Autodesk Fusion 360 part; units mm, degrees
(part 2 of 2)
sketch "Sketch6 (2)" plane through (0, -47, 0) normal (0, -1, 0) x (1, 0, 0) in component "DoserBase"
  line L0 (61.125, -2.25) -> (56.75, -2.25)
  line L1 (56.75, -2.25) -> (56.75, -6.75)
  line L2 (56.75, -6.75) -> (33, -6.75)
  line L3 (33, -6.75) -> (33, 6.75)
  line L4 (33, 6.75) -> (20, 6.75)
  line L5 (20, 6.75) -> (20, 20)
  line L6 (20, 20) -> (-10, 20)
  line L7 (-10, 20) -> (-10, -20)
  line L8 (-10, -20) -> (20, -20)
  line L9 (20, -20) -> (20, -11.75)
  line L10 (20, -11.75) -> (61.125, -11.75)
  line L11 (61.125, -11.75) -> (61.125, -2.25)
  line L12 (-7, 17) -> (17, 17)
  line L13 (17, 17) -> (17, -17)
  line L14 (17, -17) -> (-7, -17)
  line L15 (-7, -17) -> (-7, 17)
  line L16 (17, 3.75) -> (30, 3.75)
  line L17 (30, 3.75) -> (30, -8.75)
  line L18 (30, -8.75) -> (17, -8.75)
  line L19 (26.5, 15) -> (26.5, -15) construction
  line L20 (-10, 0) -> (26.5, 0) construction
  circle A0 centre (26.5, -15) radius 1.75
  circle A1 centre (26.5, 15) radius 1.75
  line L21 (20, 20) -> (33, 20)
  line L22 (33, 20) -> (33, 6.75)
  line L23 (20, -20) -> (33, -20)
  line L24 (33, -20) -> (33, -11.75)
  line L25 (33, -6.75) -> (33, -11.75) construction
  line L26 (26.5, 15) -> (26.5, 20) construction
  line L27 (-10, 20) -> (-17, 20)
  line L28 (-17, 20) -> (-17, -20)
  line L29 (-17, -20) -> (-10, -20)
  line L30 (-13.5, 20) -> (-13.5, -20) construction
  line L31 (26.5, 15) -> (-13.5, 15) construction
  line L32 (26.5, -15) -> (-13.5, -15) construction
  circle A2 centre (-13.5, 15) radius 1.75
  circle A3 centre (-13.5, -15) radius 1.75
  dimension "d242" = 3
  dimension "d243" = 3
  dimension "d244" = 3
  dimension "d245" = 3
  dimension "d246" = 3
  dimension "d247" = 3
  dimension "d248" = 3
  dimension "d254" = 30
  dimension "d257" = 3.5
  dimension "d258" = 3.5
  dimension "d260" = 3.5
  dimension "d261" = 3.5
  dimension "d262" = 40
  constraint horizontal L12
  constraint vertical L13
  constraint horizontal L14
  constraint vertical L15
  constraint coincident L13 L16.start
  constraint perpendicular L13 L16
  constraint perpendicular L16 L17
  constraint coincident L13 L18.end
  constraint perpendicular L13 L18
  constraint vertical L19
  constraint midpoint L7 L20.start
  constraint midpoint L19 L20.end
  constraint horizontal L20
  constraint coincident L19.end A0.centre
  constraint coincident L19.start A1.centre
  constraint coincident L5.end L6.start
  constraint perpendicular L5 L21
  constraint coincident L3.end L4.start
  constraint perpendicular L21 L22
  constraint coincident L8.end L9.start
  constraint perpendicular L9 L23
  constraint coincident L10 L24.end
  constraint perpendicular L10 L24
  constraint coincident L2.end L3.start
  constraint vertical L25
  constraint midpoint L21 L26.end
  constraint vertical L26
  constraint coincident L6.end L7.start
  constraint perpendicular L7 L27
  constraint perpendicular L27 L28
  constraint coincident L7.end L8.start
  constraint perpendicular L28 L29
  constraint midpoint L27 L30.start
  constraint midpoint L29 L30.end
  constraint coincident L30 L31.end
  constraint perpendicular L30 L31
  constraint coincident L30 L32.end
  constraint perpendicular L30 L32
  constraint coincident L31.end A2.centre
  constraint coincident L32.end A3.centre
  measures "d242" distance of L9 L13
  measures "d243" distance of L8 L14
  measures "d244" distance of L7 L15
  measures "d245" distance of L6 L12
  measures "d246" distance of L10 L18
  measures "d247" distance of L4 L16
  measures "d248" distance of L3 L17
  measures "d254" distance of L19.start L19.end
  measures "d257" diameter of A1
  measures "d258" diameter of A0
  measures "d260" diameter of A3
  measures "d261" diameter of A2
  measures "d262" distance of L19.start L31.end
extrude "Extrude11" cut sketch "Sketch6 (2)" against normal blind 43 contours L12 L13 L14 L15 bodies 2 in component "DoserBase"
extrude "Extrude12" cut sketch "Sketch6 (2)" against normal blind 21 contours L13 L16 L17 L18 bodies 2 in component "DoserBase"
chamfer "Chamfer2'" distance 1 angle 45 2 edges at (20, -33.15, -11.75) (20, -33.15, 6.75) on bodies 2 in component "DoserBase"
extrude "Extrude13" add sketch "Sketch6 (2)" against normal blind 3 contours L9 L10 L23 L24 | L4 L5 L21 L22 | L7 L27 L28 L29 bodies 2 in component "DoserBase"
sketch "Sketch8" plane through (-10, 0, 0) normal (-1, 0, 0) x (0, 0, 1) in component "DoserBase"
  line L0 (-20, -44) -> (20, -44)
  line L1 (20, -44) -> (20, 10.5)
  line L2 (20, 10.5) -> (11.5, 10.5)
  line L3 (11.5, 10.5) -> (11.5, 0)
  line L4 (11.5, 0) -> (-11.5, 0)
  line L5 (-11.5, 0) -> (-11.5, 10.5)
  line L6 (-11.5, 10.5) -> (-20, 10.5)
  line L7 (-20, 10.5) -> (-20, -44)
  line L8 (-20, -10) -> (20, -10) construction
  line L9 (-12.5, -5) -> (12.5, -5) construction
  line L10 (12.5, -5) -> (12.5, -15) construction
  line L11 (12.5, -15) -> (-12.5, -15) construction
  line L12 (-12.5, -15) -> (-12.5, -5) construction
  circle A0 centre (-12.5, -15) radius 0.75
  circle A1 centre (-12.5, -5) radius 0.75
  circle A2 centre (12.5, -5) radius 0.75
  circle A3 centre (12.5, -15) radius 0.75
  line L13 (0, -5) -> (0, 0) construction
  dimension "d265" = 10
  dimension "d266" = 1.5
  dimension "d267" = 1.5
  dimension "d268" = 1.5
  dimension "d269" = 1.5
  dimension "d270" = 10
  dimension "d271" = 25
  dimension "d272" = 5
  constraint coincident L7 L8.start
  constraint coincident L1 L8.end
  constraint perpendicular L1 L8
  constraint horizontal L9
  constraint vertical L10
  constraint horizontal L11
  constraint vertical L12
  constraint coincident L11.end L12.start
  constraint coincident L9.start L12.end
  constraint coincident L9.end L10.start
  constraint coincident L10.end L11.start
  constraint midpoint L9 L13.start
  constraint coincident L13.end origin
  constraint vertical L13
  measures "d265" distance of L4 L8
  measures "d266" diameter of A1
  measures "d267" diameter of A0
  measures "d268" diameter of A2
  measures "d269" diameter of A3
  measures "d270" distance of L9.start L11.end
  measures "d271" distance of L10.end L11.end
  measures "d272" distance of L8 L9
extrude "Extrude14" cut sketch "Sketch8" against normal up to surface (3 mm away) contours A0 | A1 | A2 | A3 bodies 2 in component "DoserBase"
sketch "Sketch1 (9)" plane through (-10, 0, 0) normal (-1, 0, 0) x (0, 0, 1) in component "Shoot"
  circle A0 centre (-12.5, -15) radius 0.75
  circle A1 centre (-12.5, -5) radius 0.75
  circle A2 centre (12.5, -15) radius 0.75
  circle A3 centre (12.5, -5) radius 0.75
  line L0 (-20, -44) -> (20, -44)
  line L1 (20, -44) -> (20, 10.5)
  line L2 (20, 10.5) -> (11.5, 10.5)
  line L3 (11.5, 10.5) -> (11.5, 0)
  line L4 (11.5, 0) -> (-11.5, 0)
  line L5 (-11.5, 0) -> (-11.5, 10.5)
  line L6 (-11.5, 10.5) -> (-20, 10.5)
  line L7 (-20, 10.5) -> (-20, -44)
  line L8 (-14.5, -3) -> (14.5, -3)
  line L9 (14.5, -3) -> (14.5, -17)
  line L10 (14.5, -17) -> (-14.5, -17)
  line L11 (-14.5, -17) -> (-14.5, -3)
  circle A4 centre (-12.5, -5) radius 1
  circle A5 centre (-12.5, -15) radius 1
  circle A6 centre (12.5, -15) radius 1
  circle A7 centre (12.5, -5) radius 1
  line L12 (-12.5, -5) -> (12.5, -15) construction
  line L13 (-14.5, -17) -> (14.5, -3) construction
  dimension "d279" = 2
  dimension "d280" = 2
  dimension "d281" = 2
  dimension "d282" = 2
  dimension "d283" = 14
  dimension "d284" = 29
  constraint horizontal L8
  constraint vertical L9
  constraint horizontal L10
  constraint vertical L11
  constraint concentric A1 A4
  constraint concentric A0 A5
  constraint concentric A2 A6
  constraint concentric A3 A7
  constraint coincident A1.centre A4.centre
  constraint coincident A2.centre A6.centre
  constraint midpoint L12 L13
  measures "d279" diameter of A4
  measures "d280" diameter of A5
  measures "d281" diameter of A6
  measures "d282" diameter of A7
  measures "d283" distance of L8.end L9.end
  measures "d284" distance of L9.end L10.end
extrude "Extrude1''''''''" add sketch "Sketch1 (9)" along normal blind 2 separate body contours L8 L9 L10 L11 makes body 23 in component "Shoot"
ref_plane "WorkPlane1" through (-11, -10, 0) normal (0, 1, 0) x (0, 0, -1) in component "Shoot"
sketch "Sketch3 (6)" plane through (0, -10, 0) normal (0, 1, 0) x (1, 0, 0) in component "Shoot"
  circle A0 centre (-20.25, 0) radius 8.5 construction
  circle A1 centre (-28.5, 40) radius 10
  circle A2 centre (-20.25, 0) radius 10
  line L0 (-30.0439, -2.02) -> (-38.2939, 37.98)
  line L1 (-18.7061, 42.02) -> (-10.4561, 2.02)
  line L2 (-12, -14.5) -> (-12, 14.5)
  line L3 (-12, -10) -> (-20.25, -10)
  line L4 (-10, -14.5) -> (-10, 14.5)
  line L5 (-10, 14.5) -> (-10, 50)
  line L6 (-10, 50) -> (-28.5, 50)
  line L7 (-12, -10) -> (-10, -10)
  arc A3 (-20.5, 40) -> (-36.5, 40) centre (-28.5, 40) ccw construction
  dimension "d287" = 20
  dimension "d288" = 20
  constraint concentric A1 A3
  constraint concentric A0 A2
  constraint coincident A2 L0.start
  constraint coincident A1 L0.end
  constraint tangent A1 L0
  constraint coincident A1 L1.start
  constraint coincident A2 L1.end
  constraint tangent A2 L1
  constraint tangent A2 L0
  constraint tangent A1 L1
  constraint coincident L2 L3.start
  constraint coincident A2 L3.end
  constraint tangent A2 L3
  constraint horizontal L3
  constraint coincident L4.end L5.start
  constraint parallel L4 L5
  constraint coincident A1 L6.end
  constraint tangent A1 L6
  constraint perpendicular L5 L6
  constraint coincident L4 L7.end
  constraint perpendicular L4 L7
  measures "d287" diameter of A1
  measures "d288" diameter of A2
extrude "Extrude2'''''''" add sketch "Sketch3 (6)" along normal blind -12 and the other way blind -2 bodies 23 in component "Shoot"
sketch "Sketch4 (5)" plane through (-12, 0, 0) normal (-1, 0, 0) x (0, 0, 1) in component "Shoot"
  line L0 (-14.5, -8) -> (10, -8) construction
  line L1 (10, -8) -> (10, -17) construction
  line L2 (10, -17) -> (14.5, -17) construction
  line L3 (14.5, -17) -> (14.5, -3)
  line L4 (14.5, -3) -> (-14.5, -3)
  line L5 (-14.5, -3) -> (-14.5, -8) construction
  circle A0 centre (12.5, -5) radius 1 construction
  circle A1 centre (12.5, -15) radius 1 construction
  circle A2 centre (-12.5, -5) radius 1 construction
  line L6 (14.5, -6.8072) -> (-31.5, -19)
  line L7 (-31.5, -19) -> (-30.2189, -23.8331)
  line L8 (-30.2189, -23.8331) -> (14.5, -11.9799)
  line L9 (2.02, -8) -> (-37.98, -8)
  line L10 (14.5, -17) -> (14.5, -53)
  line L11 (14.5, -53) -> (-85.5, -53)
  line L12 (-85.5, -53) -> (-85.5, -3)
  line L13 (-85.5, -3) -> (-14.5, -3)
  point P0 (10, -8)
  dimension "d291" = 5
  dimension "d292" = 17
  dimension "d293" = 11
  dimension "d294" = 100
  dimension "d295" = 50
  constraint perpendicular L6 L7
  constraint coincident L3 L8.end
  constraint perpendicular L7 L8
  constraint coincident L3 L6.start
  constraint coincident L6 P0
  constraint coincident L2.end L3.start
  constraint perpendicular L2 L10
  constraint perpendicular L10 L11
  constraint perpendicular L11 L12
  constraint coincident L4.end L5.start
  constraint perpendicular L12 L13
  measures "d291" distance of L6.end L7.end
  measures "d292" distance of L5 L6.end
  measures "d293" distance of L6.end L9
  measures "d294" distance of L10.end L11.end
  measures "d295" distance of L11.end L12.end
extrude "Extrude3'''" cut sketch "Sketch4 (5)" along normal blind 30 contours L3 L4 L6 L7 L8 L10 L11 L12 L13 bodies 23 in component "Shoot"
sketch "Sketch6 (3)" plane through (-10, 0, 0) normal (1, 0, 0) x (0, 0, -1) in component "Shoot"
  line L0 (-10, -22) -> (50, -22)
  line L1 (50, -22) -> (50, -8)
  line L2 (50, -8) -> (14.5, -8)
  line L3 (14.5, -8) -> (14.5, -3)
  line L4 (14.5, -3) -> (-14.5, -3)
  line L5 (-14.5, -3) -> (-14.5, -17)
  circle A0 centre (-12.5, -5) radius 1
  circle A1 centre (-12.5, -15) radius 1
  circle A2 centre (12.5, -5) radius 1
  line L6 (31.5, -19) -> (30.7048, -22)
  line L7 (14.5, -8) -> (14.5, -14.494)
  line L8 (-10, -8) -> (31.5, -19)
  line L9 (-10, -17) -> (-10, -22)
  line L10 (-14.5, -17) -> (-10, -17)
  constraint coincident L2.end L3.start
  constraint perpendicular L2 L7
  constraint coincident L7.end L8
extrude "Extrude5''''" cut sketch "Sketch6 (3)" against normal up to surface (2 mm away) contours L0 L1 L2 L6 L7 L8 bodies 23 in component "Shoot"
sketch "Sketch7" plane through (0, -9.9514, 2.6377) normal (0, 0.96662, -0.256213) x (-1, 0, 0) in component "Shoot"
  line L0 (36.9574, -35.3166) -> (30.0439, -0.6391)
  ellipse E0 centre (20.25, -2.7288) end of major axis (20.25, 7.6165) minor radius 10 (30.0439, -0.6391) -> (20.25, 7.6165) ccw
  line L1 (20.25, 7.6165) -> (12, 7.6165)
  line L2 (12, 7.6165) -> (12, -17.7295)
  line L3 (12, -17.7295) -> (10, -17.7295)
  line L4 (10, -17.7295) -> (10, -35.3166)
  line L5 (10, -35.3166) -> (36.9574, -35.3166)
  line L6 (34.996, -35.7076) -> (28.0825, -1.0301)
  spline S0 degree 3 poles (28.0825, -1.0301) (27.6471, 1.1538) (26.3344, 3.1212) (24.5506, 4.3078) (23.27, 5.1596) (21.7606, 5.6165) (20.25, 5.6165) knots -1.367398 -1.367398 -1.367398 -1.367398 -0.571416 -0.571416 -0.571416 0 0 0 0
  line L7 (20.25, 5.6165) -> (12, 5.6165)
  line L8 (17.5834, -35.3166) -> (12, -7.3105)
  dimension "d304" = -2
  dimension "d305" = 17
  constraint coincident L5 L8.start
  constraint parallel L6 L8
  constraint coincident L2 L8.end
  measures "d305" distance of L6 L8
extrude "Extrude6''''" cut sketch "Sketch7" against normal blind 2 contours L2 L5 L6 S0 L7 L8 bodies 23 in component "Shoot"
chamfer "Chamfer1''''" distance 4.5 distance2 5 1 edges at (-11, -17, 10) measured on face at (-10.6667, -17, 13) on bodies 23 in component "Shoot"
chamfer "Chamfer2''" distance 2 angle 45 3 edges at (-31.5002, -16.5409, -14.4166) (-25.2762, -10.9212, 6.7852) (-16.125, -10.4457, 8.5792) on bodies 23 in component "Shoot"
move_face "OffsetFaces1" offset 2 1 faces at (-15.7223, -17.2526, -22.3054) on bodies 23 in component "Shoot"
sketch "Sketch1 (10)" plane through (-43.5, 0, 0) normal (-1, 0, 0) x (0, 0, 1) in component "Component"
  line L0 (-44, -24) -> (-44, -29)
  line L1 (-44, -29) -> (-30, -29)
  line L2 (-30, -29) -> (-30, -24)
  line L3 (-30, -24) -> (-44, -24)
  circle A0 centre (-33, -26.5) radius 0.75
  line L4 (-30, -26.5) -> (-44, -26.5) construction
  line L5 (-33, -24) -> (-33, -29) construction
  circle A1 centre (-33, -26.5) radius 1.25
  line L6 (-30, -24) -> (-25, -24)
  line L7 (-30, -29) -> (-25, -29)
  line L8 (-25, -29) -> (-25, -24)
  line L9 (-50, -24) -> (-50, -23)
  line L10 (-50.5, -16) -> (-50.5, -24)
  line L11 (-50.5, -24) -> (-44, -24)
  line L12 (-50.5, -16) -> (-60.5, -16)
  line L13 (-60.5, -16) -> (-60.5, -18)
  line L14 (-60.5, -18) -> (-52.5, -18)
  line L15 (-52.5, -18) -> (-52.5, -28)
  line L16 (-52.5, -28) -> (-35, -28)
  circle A2 centre (-33, -26.5) radius 2.5
  line L17 (-25, -29) -> (-25, -34)
  line L18 (-25, -34) -> (-18, -34)
  line L19 (-18, -34) -> (-18, -44)
  line L20 (-18, -44) -> (-28, -44)
  line L21 (-28, -44) -> (-28, -29)
  line L22 (-25, -34) -> (-28, -34)
  dimension "d318" = 1.5
  dimension "d319" = 3
  dimension "d320" = 2.5
  dimension "d322" = 5
  dimension "d323" = 0.5
  dimension "d324" = 2
  dimension "d325" = 2
  dimension "d326" = 8
  dimension "d327" = 10
  dimension "d328" = 4
  dimension "d335" = 3
  dimension "d336" = 10
  dimension "d337" = 10
  dimension "d338" = 15
  constraint midpoint L2 L4.start
  constraint midpoint L0 L4.end
  constraint coincident L3 L5.start
  constraint coincident L1 L5.end
  constraint perpendicular L1 L5
  constraint midpoint A0.centre L5
  constraint concentric A0 A1
  constraint coincident L2.end L3.start
  constraint perpendicular L2 L6
  constraint coincident L1.end L2.start
  constraint perpendicular L2 L7
  constraint perpendicular L6 L8
  constraint parallel L9 L10
  constraint coincident L0.start L3.end
  constraint perpendicular L10 L11
  constraint perpendicular L10 L12
  constraint perpendicular L12 L13
  constraint perpendicular L13 L14
  constraint perpendicular L14 L15
  constraint perpendicular L15 L16
  constraint concentric A1 A2
  constraint coincident L5.end A2
  constraint coincident L16.end A2
  constraint perpendicular L7 L17
  constraint perpendicular L8 L18
  constraint perpendicular L7 L19
  constraint perpendicular L8 L20
  constraint coincident L7 L21.end
  constraint perpendicular L7 L21
  constraint coincident L21 L22.end
  constraint perpendicular L21 L22
  measures "d318" diameter of A0
  measures "d319" distance of L2 L5
  measures "d320" diameter of A1
  measures "d322" distance of L1.end L7.end
  measures "d323" distance of L9 L10
  measures "d324" distance of L10 L15
  measures "d325" distance of L12 L14
  measures "d326" distance of L10.start L10.end
  measures "d327" distance of L10.start L12.end
  measures "d328" distance of L11 L16
  measures "d335" distance of L17 L21
  measures "d336" distance of L18.end L19.end
  measures "d337" distance of L19.end L20.end
  measures "d338" distance of L20.end L21.end
extrude "Extrude1'''''''''" add sketch "Sketch1 (10)" along normal blind 2 separate body contours L0 L3 L16 A2 | L0 L10 L11 L12 L13 L14 L15 L16 | L1 L2 L3 A2 | A2 | L2 L6 L7 L8 | L7 L17 L21 L22 | L18 L19 L20 L21 L22 makes body 24 in component "Component"
sketch "Sketch2 (9)" plane through (-43.5, 0, 0) normal (1, 0, 0) x (0, 0, -1) in component "Component"
  circle A0 centre (33, -26.5) radius 1.25
  line L0 (60.5, -16) -> (50.5, -16)
  line L1 (50.5, -16) -> (50.5, -24)
  line L2 (50.5, -24) -> (25, -24)
  line L3 (25, -24) -> (25, -34)
  line L4 (28, -29) -> (33, -29)
  arc A1 (33, -29) -> (35, -28) centre (33, -26.5) ccw
  line L5 (35, -28) -> (52.5, -28)
  line L6 (52.5, -28) -> (52.5, -18)
  line L7 (52.5, -18) -> (60.5, -18)
  line L8 (60.5, -18) -> (60.5, -16)
  line L9 (50.5, -24) -> (50.5, -28)
  line L10 (25, -34) -> (18, -34)
  line L11 (18, -34) -> (18, -44)
  line L12 (18, -44) -> (28, -44)
  line L13 (28, -44) -> (28, -29)
  constraint coincident L1.end L2.start
  constraint coincident L5 L9.end
  constraint perpendicular L5 L9
extrude "Extrude2''''''''" add sketch "Sketch2 (9)" along normal blind 25 contours L0 L1 L5 L6 L7 L8 L9 bodies 24 in component "Component"
extrude "Extrude7'''" cut sketch "Sketch1 (10)" against normal up to surface (4.5 mm away) contours A0 sketch seen with x (1, 0, 0) y (0, 1, 0) z (0, 0, 1) at (28.5, 47, 40) bodies 19 in component "SensorStand"
extrude "Extrude3''''" add sketch "Sketch1 (10)" against normal blind 20 contours L18 L19 L20 L21 L22 bodies 24 in component "Component"
chamfer "Chamfer1'''''" distance 8 angle 45 1 edges at (-44.5, -24, -50.5) on bodies 24 in component "Component"
fillet "Fillet1'''''" radius 3 1 edges at (-44.5, -24, -25) on bodies 24 in component "Component"
fillet "Fillet2'" radius 2 1 edges at (-44.5, -29, -28) on bodies 24 in component "Component"
fillet "Fillet3" radius 5 2 edges at (-15, 23.5, -10) (15, 23.5, -10) on bodies 20 in component "SensorPlate"
chamfer "Chamfer2'''" distance 4 angle 45 1 edges at (-43.5, -34, -26.5) on bodies 24 in component "Component"
fillet "Fillet3'" radius 5.5 1 edges at (-43.5, -22, -50.5) on bodies 24 in component "Component"
sketch "Sketch3 (7)" plane through (-23.5, 0, 0) normal (1, 0, 0) x (0, 0, -1) in component "Component"
  line L0 (28, -34) -> (18, -34)
  line L1 (18, -34) -> (18, -44)
  line L2 (18, -44) -> (28, -44)
  line L3 (28, -44) -> (28, -34)
  line L4 (27, -43) -> (27, -35)
  line L5 (27, -35) -> (19, -35)
  line L6 (19, -35) -> (19, -43)
  line L7 (19, -43) -> (27, -43)
  dimension "d357" = -1
extrude "Extrude4'''''" cut sketch "Sketch3 (7)" against normal blind 20 contours L4 L5 L6 L7 bodies 24 in component "Component"
fillet "Fillet4" radius 1 4 edges at (-34.5, -34, -18) (-34.5, -44, -18) (-31.5, -34, -28) (-34.5, -44, -28) on bodies 24 in component "Component"
fillet "Fillet5" radius 2 2 edges at (-45.5, -17, -60.5) (-18.5, -17, -60.5) on bodies 24 in component "Component"
sketch "Sketch4 (6)" plane through (-43.5, 0, 0) normal (1, 0, 0) x (0, 0, -1) in component "Component"
  line L0 (45, -28) -> (45, -21.5)
  line L1 (45, -21.5) -> (42.5, -24)
  line L2 (42.5, -24) -> (28, -24)
  arc A0 (28, -24) -> (25, -27) centre (28, -27) ccw
  line L3 (25, -27) -> (25, -30)
  line L4 (25, -30) -> (28.2679, -30)
  arc A1 (30, -29) -> (28.2679, -30) centre (30, -31) ccw
  line L5 (30, -29) -> (33, -29)
  arc A2 (33, -29) -> (35, -28) centre (33, -26.5) ccw
  line L6 (35, -28) -> (45, -28)
  circle A3 centre (33, -26.5) radius 1.25
  circle A4 centre (33, -26.5) radius 2.5
  constraint concentric A2 A4
  constraint tangent L2 A4
extrude "Extrude5'''''" add sketch "Sketch4 (6)" along normal blind 0.5 contours A2 A4 bodies 24 in component "Component"
sketch "Sketch6 (4)" plane through (0, 3, 0) normal (0, 1, 0) x (-1, 0, 0) in component "SensorStand"
  line L0 (-10, -4) -> (-10, 10)
  line L1 (-10, 10) -> (-20, 10)
  line L2 (-20, 10) -> (-20, -10)
  line L3 (-20, -10) -> (20, -10)
  line L4 (20, -10) -> (20, 10)
  line L5 (20, 10) -> (10, 10)
  line L6 (10, 10) -> (10, -4)
  line L7 (10, -4) -> (-10, -4)
  circle A0 centre (15, -5) radius 1.5
  circle A1 centre (-15, -5) radius 1.5
  circle A2 centre (-15, 5) radius 1.5
  circle A3 centre (15, 5) radius 1.5
  line L8 (-10, -4) -> (-10, -10)
  line L9 (10, -4) -> (10, -10)
  constraint coincident L0.start L7.end
  constraint coincident L3 L8.end
  constraint perpendicular L3 L8
  constraint coincident L6.end L7.start
  constraint coincident L3 L9.end
  constraint perpendicular L3 L9
extrude "Extrude8'" cut sketch "Sketch6 (4)" against normal up to surface (3 mm away) contours L3 L7 L8 L9 bodies 19 in component "SensorStand"
chamfer "Chamfer2''''" distance 2 angle 45 2 edges at (-10, 1.5, -4) (10, 1.5, -4) on bodies 19 in component "SensorStand"
sketch "Sketch7 (2)" plane through (0, 0, -4) normal (0, 0, -1) x (-1, 0, 0) in component "SensorStand"
  line L0 (-8, 3) -> (-8, 0)
  line L1 (-8, 0) -> (8, 0)
  line L2 (8, 0) -> (8, 3)
  line L3 (8, 3) -> (10, 3)
  line L4 (10, 3) -> (10, 8)
  line L5 (10, 8) -> (15, 18)
  line L6 (15, 18) -> (15, 23)
  line L7 (15, 23) -> (10.5, 23)
  line L8 (10.5, 23) -> (10.5, 20)
  line L9 (10.5, 20) -> (-10.5, 20)
  line L10 (-10.5, 20) -> (-10.5, 23)
  line L11 (-10.5, 23) -> (-15, 23)
  line L12 (-15, 23) -> (-15, 18)
  line L13 (-15, 18) -> (-10, 8)
  line L14 (-10, 8) -> (-10, 3)
  line L15 (-10, 3) -> (-8, 3)
  line L16 (2, 5) -> (2, 0)
  line L17 (-2, 0) -> (-2, 5)
  line L18 (0, 5) -> (0, 0) construction
  circle A0 centre (0, 5) radius 2
  dimension "d369" = 4
  dimension "d370" = 5
  constraint vertical L16
  constraint vertical L17
  constraint coincident L18.end origin
  constraint coincident L18.start A0.centre
  constraint coincident L16.start A0
  constraint coincident L17.end A0
  constraint tangent L17 A0
  constraint coincident L1 L17.start
  constraint coincident L1 L16.end
  constraint tangent L16 A0
  constraint vertical L18
  measures "d369" distance of L16 L17
  measures "d370" vertical distance of L18.start L18.end
extrude "Extrude9'" cut sketch "Sketch7 (2)" against normal up to surface (14 mm away) contours L1 L16 L17 A0 | A0 bodies 19 in component "SensorStand"
component "DoserSlider" placed x (1, 0, 0) y (0, 1, 0) z (0, 0, 1) at (-0.25, 0.25, 0)
component "DoserBase" placed x (1, 0, 0) y (0, 1, 0) z (0, 0, 1) at (0, 0, 0)
component "Hopper" placed x (1, 0, 0) y (0, 1, 0) z (0, 0, 1) at (0, 0, 0)
component "SensorPCB" placed x (1, 0, 0) y (0, 1, 0) z (0, 0, 1) at (-28.5, -27, -40)
component "SensorStand" placed x (1, 0, 0) y (0, 1, 0) z (0, 0, 1) at (-28.5, -47, -40)
component "SensorPlate" placed x (1, 0, 0) y (0, 1, 0) z (0, 0, 1) at (-28.5, -47, -40)
component "Srevo_MG90S" placed x (-1, 0, 0) y (0, 1, 0) z (0, 0, -1) at (44.875, -16.2, 0)
component "SliderSwing" placed x (1, 0, 0) y (0, 1, 0) z (0, 0, 1) at (50, -7, 0)
component "Shoot" placed x (1, 0, 0) y (0, 1, 0) z (0, 0, 1) at (0, 0, 0)
component "Component" placed x (1, 0, 0) y (0, 1, 0) z (0, 0, 1) at (-0.5, 0, 0)
equation "d19 = d13"
equation "d30 = d29"
equation "d58 = d57"
equation "d60 = d59"
equation "d109 = d108"
equation "d110 = d108"
equation "d111 = d108"
equation "d115 = 20 mm - 3 mm"
equation "d122 = d121"
equation "d124 = d121"
equation "d134 = d133"
equation "d138 = d137"
equation "d140 = d139"
equation "d207 = d206 / 2"
equation "d231 = d230"
equation "d243 = d242"
equation "d244 = d242"
equation "d245 = d242"
equation "d246 = d242"
equation "d247 = d242"
equation "d248 = d242"
equation "d258 = d257"
equation "d260 = d257"
equation "d261 = d257"
equation "d267 = d266"
equation "d268 = d266"
equation "d269 = d266"
equation "d280 = d279"
equation "d281 = d279"
equation "d282 = d279"
equation "d325 = d324"
